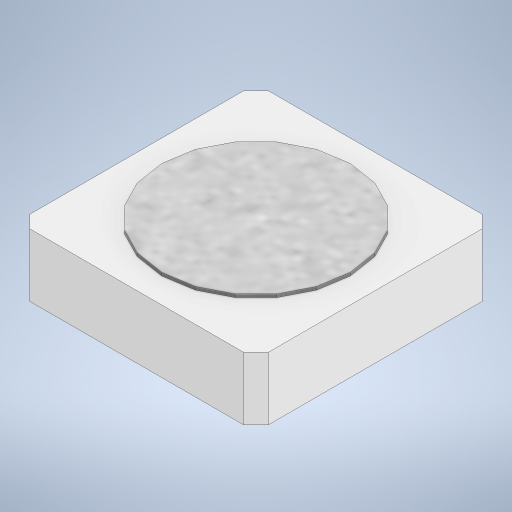
# Autodesk Inventor part: 樓上跟尖下
Saved by Autodesk Inventor 2024.2 (Build 282272000, 272)
## iProperties
Created: 2024-06-04
Part Number: 樓上跟尖下
Material: 一般
Document SubType Name: Modeling
Designer: sohil
Density: 1 g/cm^3
Appearance: 預設
Author: sohil
Autodesk Inventor part; units mm, degrees
ref_plane "YZ Plane" through (0, 0, 0) normal (1, 0, 0) x (0, 1, 0)
ref_plane "XZ Plane" through (0, 0, 0) normal (0, 1, 0) x (-1, 0, 0)
ref_plane "XY Plane" through (0, 0, 0) normal (0, 0, 1) x (1, 0, 0)
sketch "草圖1" plane through (0, 0, 0) normal (0, 1, 0) x (-1, 0, 0)
  line L0 (0, 0) -> (-35, 0)
  line L1 (-35, 0) -> (-35, -40)
  line L2 (-35, -40) -> (0, -40)
  line L3 (0, -40) -> (0, 0)
  line L4 (0, -40) -> (0, -39)
  line L5 (0, -39) -> (-35, -39)
  line L6 (-35, -39) -> (-35, -40)
  line L7 (-35, -40) -> (0, -40)
  line L8 (0, 0) -> (0, -1)
  line L9 (0, -1) -> (-35, -1)
  line L10 (-35, -1) -> (-35, 0)
  line L11 (-35, 0) -> (0, 0)
  dimension "d0" = 35
  dimension "d1" = 40
  dimension "d19" = 1
  dimension "d20" = 1
  constraints: 24 end point, 6 parallel, 3 perpendicular, 2 point on line, 1 horizontal
  measures "d0" distance of L2.end L1.end
  measures "d1" distance of L2.end L0.start
  measures "d19" distance of L2.end L4.end
  measures "d20" distance of L0.start L8.end
extrude "擠出1" add sketch "草圖1" along normal blind 10 contours L3 L5 L1 L9
sketch "草圖2" plane through (0, 10, 0) normal (0, 1, 0) x (1, 0, 0)
  line L0 (0, 0) -> (0, 20)
  line L1 (0, 20) -> (17.5, 20)
  line L2 (17.5, 20) -> (17.5, 0)
  line L3 (17.5, 0) -> (0, 0)
  line L4 (17.5, 20) -> (2.5, 20)
  line L5 (2.5, 20) -> (3.2342, 24.6353)
  line L6 (3.2342, 24.6353) -> (5.3647, 28.8168)
  line L7 (5.3647, 28.8168) -> (8.6832, 32.1353)
  line L8 (8.6832, 32.1353) -> (12.8647, 34.2658)
  line L9 (12.8647, 34.2658) -> (17.5, 35)
  line L10 (17.5, 35) -> (22.1353, 34.2658)
  line L11 (22.1353, 34.2658) -> (26.3168, 32.1353)
  line L12 (26.3168, 32.1353) -> (29.6353, 28.8168)
  line L13 (29.6353, 28.8168) -> (31.7658, 24.6353)
  line L14 (31.7658, 24.6353) -> (32.5, 20)
  line L15 (32.5, 20) -> (31.7658, 15.3647)
  line L16 (31.7658, 15.3647) -> (29.6353, 11.1832)
  line L17 (29.6353, 11.1832) -> (26.3168, 7.8647)
  line L18 (26.3168, 7.8647) -> (22.1353, 5.7342)
  line L19 (22.1353, 5.7342) -> (17.5, 5)
  line L20 (17.5, 5) -> (12.8647, 5.7342)
  line L21 (12.8647, 5.7342) -> (8.6832, 7.8647)
  line L22 (8.6832, 7.8647) -> (5.3647, 11.1832)
  line L23 (5.3647, 11.1832) -> (3.2342, 15.3647)
  line L24 (3.2342, 15.3647) -> (2.5, 20)
  dimension "d7" = 17.5
  dimension "d8" = 20
  dimension "d9" = 15
  constraints: 50 end point, 2 parallel, 1 coincident, 1 perpendicular, 1 point on line, 1 vertical, 41 other
  measures "d7" distance of L0.end L1.end
  measures "d8" distance of L0.start L0.end
  measures "d9" distance of L1.end L4.end
extrude "擠出2" add sketch "草圖2" along normal blind 0.5 contours L5 L6 L7 L8 L9 L10 L11 L12 L13 L14 L15 L16 L17 L18 L19 L2 L1 | L1 L2 L20 L21 L22 L23 L24
sketch "草圖3" plane through (35, 0, 0) normal (1, 0, 0) x (0, 0, -1)
  line L0 (40, 0) -> (40, 10) projected
  line L1 (1, 10) -> (39, 10) projected
  line L2 (40, 0) -> (40, 10)
  line L3 (40, 10) -> (0, 10)
  line L4 (0, 10) -> (0, 0)
  line L5 (0, 0) -> (40, 0)
  line L6 (1, 0) -> (1, 10) projected
  line L7 (0, 10) -> (1, 10)
  line L8 (1, 10) -> (1, 0)
  line L9 (1, 0) -> (0, 0)
  line L10 (0, 0) -> (0, 10)
  line L11 (39, 0) -> (39, 10) projected
  line L12 (39, 10) -> (40, 10)
  line L13 (40, 10) -> (40, 0)
  line L14 (40, 0) -> (39, 0)
  line L15 (39, 0) -> (39, 10)
  point P0 (0, 0)
  constraints: 24 end point, 6 parallel, 4 perpendicular, 1 collinear, 1 vertical
extrude "擠出3" add sketch "草圖3" along normal blind 1.5 contours L5 L6 L1 L11
sketch "草圖4" plane through (0, 0, -40) normal (-1, 0, 0) x (0, 0, 1)
  line L0 (0, 10) -> (40, 10)
  line L1 (40, 10) -> (40, 0)
  line L2 (40, 0) -> (0, 0)
  line L3 (0, 0) -> (0, 10)
  line L4 (1, 0) -> (1, 10) projected
  line L5 (1, 0) -> (1, 10)
  line L6 (39, 0) -> (39, 10) projected
  line L7 (1, 10) -> (39, 10)
  line L8 (39, 10) -> (39, 0)
  line L9 (0, 10) -> (1, 10)
  line L10 (1, 10) -> (1, 0)
  line L11 (1, 0) -> (0, 0)
  line L12 (0, 0) -> (0, 10)
  line L13 (39, 10) -> (40, 10)
  line L14 (40, 10) -> (40, 0)
  line L15 (40, 0) -> (39, 0)
  line L16 (39, 0) -> (39, 10)
  constraints: 30 end point, 6 parallel, 6 perpendicular, 2 collinear
extrude "擠出4" add sketch "草圖4" along normal blind 1.5 contours L0 L6 L2 L4
chamfer "倒角3" distance 2 angle 45 4 edges at (36.5, 5, -1) (36.5, 5, -39) (-1.5, 5, -39) (-1.5, 5, -1)
